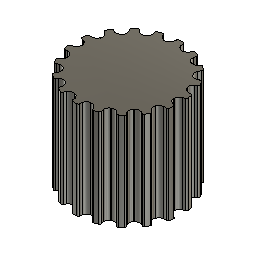
gear_18z (Autodesk Fusion 360 design; units mm, degrees)
Autodesk Fusion 360 part; units mm, degrees
note: some values were not read from the file. Set by a fixed rule: which sketch regions a step uses.
sketch "Sketch1" plane through (0, 0, 0) normal (0, 0, 1) x (1, 0, 0) in component "gt2 pulley"
  circle A0 centre (0, 0) radius 5.7296 construction
  circle A1 centre (0, 0) radius 4.7256 construction
  line L0 (0, 0) -> (0, 5.7296) construction
  line L1 (0, 0) -> (0.9949, 5.6425) construction
  line L2 (0, 0) -> (1.4116, 5.553) construction
  circle A2 centre (0, 0) radius 5.4756 construction
  arc A3 (0.3491, 5.3199) -> (0.3781, 5.0676) centre (1.349, 5.3068) ccw
  circle A4 centre (0, 0) radius 5.3256 construction
  arc A5 (0.2047, 5.4718) -> (0, 5.4756) centre (0, 0) ccw
  arc A6 (0.3491, 5.3199) -> (0.2047, 5.4718) centre (0.1991, 5.3219) ccw
  arc A7 (0.3781, 5.0676) -> (0.8206, 4.6538) centre (0.917, 5.2004) ccw
  arc A8 (0, 5.4756) -> (-0.2047, 5.4718) centre (0, 0) ccw
  arc A9 (-0.2047, 5.4718) -> (-0.3491, 5.3199) centre (-0.1991, 5.3219) ccw
  arc A10 (-0.3781, 5.0676) -> (-0.3491, 5.3199) centre (-1.349, 5.3068) ccw
  arc A11 (-0.8206, 4.6538) -> (-0.3781, 5.0676) centre (-0.917, 5.2004) ccw
  arc A12 (0.8206, 4.6538) -> (-0.8206, 4.6538) centre (0, 0) ccw
  point P0 (1.349, 5.3068)
  point P1 (0, 5.4756)
  dimension "d18" = 11.4592
  dimension "d19" = 10
  dimension "d22" = 1.004
  dimension "d24" = 0.75
  dimension "d26" = 1
  dimension "d27" = 0.15
  dimension "d28" = 0.15
  dimension "d47" = 0.555
  dimension "d52" = 3.812
  constraint coincident A0.centre A1.centre
  constraint coincident A0 L0.end
  constraint vertical L0
  constraint coincident A0 L1.end
  constraint coincident A0 L2.end
  constraint concentric A1 A2
  constraint coincident A1 A7.end
  constraint coincident L1 A7.end
  constraint coincident A2 P0
  constraint coincident L2 P0
  constraint coincident P0 A3.centre
  constraint coincident A2 P1
  constraint coincident L0 P1
  constraint concentric A2 A4
  constraint coincident P1 A5.end
  constraint coincident A4 A6.centre
  constraint coincident A3.start A6.start
  constraint tangent A3 A6
  constraint tangent A3 A7
  constraint symmetric L0 A7.end A11.start
  constraint symmetric L0 A3.start A9.end
  constraint symmetric L0 A3.end A10.start
  constraint symmetric L0 A3 A10
  constraint symmetric L0 A5.start A8.end
  constraint symmetric L0 P1 A5.end
  constraint symmetric L0 A5 A8
  constraint symmetric L0 A6 A9
  constraint symmetric L0 A7 A11
  constraint coincident A1 A11.start
  constraint tangent A1 A7
  constraint coincident L1 A7.centre
  measures "d18" diameter of A0
  measures "d19" angle of L0 L1
  measures "d22" distance of A0 A1
  measures "d24" distance of A1 A2
  measures "d26" radius of A3
  measures "d27" distance of A2 A4
  measures "d28" radius of A6
  measures "d47" radius of A7
extrude "Extrude1" add sketch "Sketch1" along normal blind 10 makes body 1
pattern_circular "C-Pattern1" count 18 over 360 about axis through (0, 0, 1.75) along (0, 0, 1) of bodies 1 makes body 2 at (-1.702, 4.4084, 6.6667) makes body 3 at (-3.4995, 3.1756, 6.6667) makes body 4 at (-4.1375, 2.283, 6.6667) makes body 5 at (-4.4999, 1.4428, 3.3333) makes body 6 at (-4.637, -0.9107, 6.6667) makes body 7 at (-4.0459, -2.4417, 6.6667) makes body 8 at (-2.5197, -3.9978, 6.6667) makes body 9 at (-2.2023, -4.181, 3.3333) makes body 10 at (0.0916, -4.7247, 6.6667) makes body 11 at (1.0004, -4.6185, 3.3333) makes body 12 at (3.1072, -3.5604, 6.6667) makes body 13 at (4.1375, -2.283, 6.6667) makes body 14 at (4.4999, -1.4428, 3.3333) makes body 15 at (4.637, 0.9107, 6.6667) makes body 16 at (4.0459, 2.4417, 6.6667) makes body 17 at (3.4995, 3.1756, 3.3333) makes body 18 at (1.5298, 4.4711, 6.6667)
sketch "Sketch2" plane through (0, 0, 10) normal (0, 0, 1) x (-1, 0, 0)
  arc A0 (1.4914, -5.1185) -> (1.6791, -5.2118) centre (1.633, -5.069) ccw
  arc A1 (1.6791, -5.2118) -> (2.0638, -5.0718) centre (0, 0) ccw
  arc A2 (2.0638, -5.0718) -> (2.1476, -4.8796) centre (2.0073, -4.9328) ccw
  arc A3 (2.0885, -4.6327) -> (2.1476, -4.8796) centre (3.0827, -4.5254) ccw
  arc A4 (2.3628, -4.0925) -> (2.0885, -4.6327) centre (2.6403, -4.5731) ccw
  arc A5 (0.8206, -4.6538) -> (2.3628, -4.0925) centre (0, 0) ccw
  arc A6 (1.378, -4.8913) -> (0.8206, -4.6538) centre (0.917, -5.2004) ccw
  arc A7 (1.4914, -5.1185) -> (1.378, -4.8913) centre (0.5473, -5.4482) ccw
  circle A8 centre (0, 0) radius 4.7262
  constraint concentric A1 A8
extrude "Extrude2" add sketch "Sketch2" against normal blind 10 contours A5 A8 bodies 1 2 3 4 5 6 7 8 9 10 11 12 13 14 15 16 17 18
extrude "Extrude4" [suppressed] in component "gt2 pulley"
pattern_circular "C-Pattern7" [suppressed] in component "gt2 pulley"
extrude "Extrude3" [suppressed] in component "gt2 pulley"
pattern_circular "C-Pattern6" [suppressed] in component "gt2 pulley"
extrude "Extrude2'" [suppressed] in component "gt2 pulley"
pattern_circular "C-Pattern5" [suppressed] in component "gt2 pulley"
extrude "Extrude1'" [suppressed] in component "gt2 pulley"
pattern_circular "C-Pattern4" [suppressed] in component "gt2 pulley"
pattern_circular "C-Pattern3" [suppressed] in component "gt2 pulley"
pattern_circular "C-Pattern2" [suppressed] in component "gt2 pulley"
pattern_circular "C-Pattern1'" [suppressed] in component "gt2 pulley"
copy_body "Body->Comp1" [suppressed] in component "Component"
copy_body "Body->Comp2" [suppressed] in component "Component'"
copy_body "Body->Comp3" [suppressed] in component "Component''"
copy_body "Body->Comp4" [suppressed] in component "Component'''"
copy_body "Body->Comp5" [suppressed] in component "Component''''"
copy_body "Body->Comp6" [suppressed] in component "Component'''''"
copy_body "Body->Comp7" [suppressed] in component "Component''''''"
copy_body "Body->Comp8" [suppressed] in component "Component'''''''"
copy_body "Body->Comp9" [suppressed] in component "Component''''''''"
copy_body "Body->Comp10" [suppressed] in component "Component'''''''''"
copy_body "Body->Comp11" [suppressed] in component "Component''''''''''"
copy_body "Body->Comp12" [suppressed] in component "Component'''''''''''"
copy_body "Body->Comp13" [suppressed] in component "Component''''''''''''"
copy_body "Body->Comp14" [suppressed] in component "Component'''''''''''''"
copy_body "Body->Comp15" [suppressed] in component "Component''''''''''''''"
copy_body "Body->Comp16" [suppressed] in component "Component'''''''''''''''"
copy_body "Body->Comp17" [suppressed] in component "Component''''''''''''''''"
copy_body "Body->Comp18" [suppressed] in component "Component'''''''''''''''''"
copy_body "Body->Comp19" [suppressed] in component "Component''''''''''''''''''"
copy_body "Body->Comp20" [suppressed] in component "Component'''''''''''''''''''"
component "gt2 pulley" placed x (1, 0, 0) y (0, 1, 0) z (0, 0, 1) at (0, 0, 0)
equation "NumTeeth = 18" comment "min 20"
equation "ToothPitch = 2 mm"
equation "PullyDia = NumTeeth * ToothPitch / PI"
equation "ToothAng = ( ( 360 / NumTeeth ) * 1 deg )"
equation "TransOffsetAngle = ToothAng * 0.2"
equation "Sholulder_Radius = 0.15 mm"
equation "Root_Radius = 0.555 mm"
equation "TransRadius = 1 mm"
equation "ToolHeight = 0.75 mm"
equation "PLD = 0.254 mm"
equation "d18 = PullyDia"
equation "d19 = ToothAng / 2"
equation "d22 = PLD + ToolHeight"
equation "d24 = ToolHeight"
equation "d26 = TransRadius"
equation "d27 = Sholulder_Radius"
equation "d31 = NumTeeth"
equation "d33 = NumTeeth"
equation "d35 = NumTeeth"
equation "d37 = NumTeeth"
equation "d41 = NumTeeth"
equation "d45 = NumTeeth"
equation "d47 = Root_Radius"
equation "d50 = NumTeeth"
